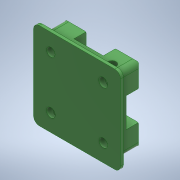
# Autodesk Inventor part: 071_0100_Base
Saved by Autodesk Inventor 2020 (Build 240168000, 168)
## iProperties
Created: 2018-07-06
Part Number: 071_0100_Base
Material: Generic
Document SubType Name: Modeling
Designer: deniz
Density: 1 g/cm^3
Appearance: Default
d_clamp_total: 51.477 mm
d_clamp_center: 25.739 mm
d_bottom_length: 52.400 mm
Author: deniz
Autodesk Inventor part; units mm, degrees
ref_plane "YZ Plane" through (0, 0, 0) normal (1, 0, 0) x (0, 1, 0)
ref_plane "XZ Plane" through (0, 0, 0) normal (0, 1, 0) x (-1, 0, 0)
ref_plane "XY Plane" through (0, 0, 0) normal (0, 0, 1) x (1, 0, 0)
sketch "Sketch1" plane through (0, 0, 0) normal (0, 1, 0) x (-1, 0, 0)
  line L0 (0, 0) -> (30, 0)
  line L1 (30, 0) -> (30, -30)
  line L2 (30, -30) -> (0, -30)
  line L3 (0, -30) -> (0, 0)
  line L4 (30, 0) -> (0, -30) construction
  line L5 (0, 0) -> (30, -30) construction
  line L6 (25.2, 0) -> (25.2, -4.8)
  line L7 (25.2, -4.8) -> (30, -4.8)
  line L8 (25.2, -25.2) -> (25.2, -30)
  line L9 (25.2, -25.2) -> (30, -25.2)
  line L10 (4.8, -25.2) -> (0, -25.2)
  line L11 (4.8, -25.2) -> (4.8, -30)
  line L12 (4.8, -4.8) -> (4.8, 0)
  line L13 (4.8, -4.8) -> (0, -4.8)
  line L14 (41.2, 11.2) -> (-11.2, 11.2)
  line L15 (-11.2, 11.2) -> (-11.2, -41.2)
  line L16 (-11.2, -41.2) -> (41.2, -41.2)
  line L17 (41.2, -41.2) -> (41.2, 11.2)
  circle A0 centre (33.2, 3.2) radius 5 construction
  line L18 (25.2, 0) -> (25.2, 11.2)
  line L19 (30, -4.8) -> (41.2, -4.8)
  line L20 (4.8, 0) -> (4.8, 11.2)
  line L21 (0, -4.8) -> (-11.2, -4.8)
  line L22 (0, -25.2) -> (-11.2, -25.2)
  line L23 (4.8, -30) -> (4.8, -41.2)
  line L24 (25.2, -30) -> (25.2, -41.2)
  line L25 (30, -25.2) -> (41.2, -25.2)
  line L26 (33.2, 3.2) -> (-3.2, -33.2) construction
  line L27 (33.2, 3.2) -> (-3.2, 3.2) construction
  line L28 (-3.2, 3.2) -> (-3.2, -33.2) construction
  line L29 (-3.2, -33.2) -> (33.2, -33.2) construction
  line L30 (33.2, -33.2) -> (33.2, 3.2) construction
  circle A1 centre (56.9794, 13.0498) radius 7.5
  arc A2 (58.5888, -1.0296) -> (56.9794, 13.0498) centre (33.2, 3.2) ccw construction
  arc A3 (62.0412, -1.6047) -> (60.213, 14.3892) centre (33.2, 3.2) ccw
  arc A4 (55.1364, -0.4544) -> (53.7459, 11.7104) centre (33.2, 3.2) ccw
  arc A5 (55.1364, -0.4544) -> (62.0412, -1.6047) centre (58.5888, -1.0296) ccw
  arc A6 (60.213, 14.3892) -> (53.7459, 11.7104) centre (56.9794, 13.0498) ccw
  line L31 (56.9794, 13.0498) -> (33.2, 3.2) construction
  point P0 (15, -15)
  dimension "d0" = 30
  dimension "d1" = 30
  dimension "d2" = 20.4
  dimension "d13" = 10
  dimension "d_clamp_total" = 51.4774
  dimension "d_clamp_center" = 25.7387
  dimension "d_bottom_length" = 52.4
  dimension "d52" = 8
  dimension "d53" = 8
  dimension "d54" = 8
  dimension "d55" = 8
  dimension "d56" = 8
  dimension "d58" = 15
  dimension "d59" = 7
  dimension "d61" = 22.5
  dimension "d62" = 25.7387
  dimension "d73" = 8
  dimension "d74" = 8
  constraints: 64 end point, 31 point on line, 10 perpendicular, 10 point on circle, 7 centre point, 6 coincident, 6 parallel, 4 tangent, 3 horizontal, 2 midpoint, 1 vertical
  measures "d0" distance of L1.end L2.end
  measures "d1" distance of L0.end L1.end
  measures "d2" distance between parallel lines of L9 L7
  measures "d13" diameter of A0
  measures "d_clamp_total" distance of L26.start L26.end
  measures "d_clamp_center" distance of point (15, -15) A0.centre
  measures "d_bottom_length" distance between parallel lines of L15 L17
  measures "d52" distance between parallel lines of L15 L28
  measures "d53" distance between parallel lines of L16 L29
  measures "d54" distance between parallel lines of L14 L27
  measures "d55" distance between parallel lines of L17 L30
  measures "d56" distance between parallel lines of L24 L30
  measures "d58" diameter of A1
  measures "d59" diameter of A5
  measures "d61" angle of L27 L31
  measures "d62" distance of L31.start L26.start
  measures "d73" distance from line of L26.end L23
  measures "d74" distance from line of L22 L26.end
extrude "Extrusion1" add sketch "Sketch1" along normal blind 2 contours L20 L14 L18 L0 | L0 L6 L7 L1 L9 L8 L2 L11 L10 L3 L13 L12 | L3 L22 L15 L21 | L19 L17 L25 L1 | L2 L24 L16 L23
extrude "Extrusion2" add sketch "Sketch1" along normal blind 12 contours L3 L21 L15 L14 L20 L0 | L0 L12 L13 L3 | L18 L14 L17 L19 L1 L0 | L0 L1 L7 L6 | L10 L11 L2 L3 | L3 L2 L23 L16 L15 L22 | L25 L17 L16 L24 L2 L1 | L1 L2 L8 L9
hole "Hole1" at (-33.2, 0, -33.2) at (3.2, 0, 3.2) direction (0, 1, 0) diameter 6.2 depth 20 tip angle 118 start extended yes
hole "Hole2" at (3.2, 0, -33.2) at (-33.2, 0, 3.2) direction (0, 1, 0) diameter 5.9 depth 20 tip angle 118 start extended yes
sketch "Sketch2" plane through (0, 12, 0) normal (0, 1, 0) x (1, 0, 0)
  circle A0 centre (-56.9794, -13.0498) radius 7.5 projected
  point P0 (0, 0)
extrude "Extrusion4" [suppressed]
sketch "Sketch3" plane through (-56.9794, 18, 13.0498) normal (0, 1, 0) x (1, 0, 0)
  circle A0 centre (60.1794, 46.2498) radius 2.95 projected
  circle A1 centre (23.7794, 9.8498) radius 2.95 projected
  circle A2 centre (23.7794, 46.2498) radius 3.1 projected
  circle A3 centre (60.1794, 9.8498) radius 3.1 projected
  line L0 (15.7794, 54.2498) -> (15.7794, 1.8498) projected
  line L1 (68.1794, 54.2498) -> (15.7794, 54.2498) projected
  line L2 (68.1794, 1.8498) -> (68.1794, 54.2498) projected
  line L3 (15.7794, 1.8498) -> (68.1794, 1.8498) projected
  arc A4 (1.8431, 13.5042) -> (-5.0618, 14.6545) centre (-1.6093, 14.0793) ccw projected
  arc A5 (-5.0618, 14.6545) -> (-3.2336, -1.3394) centre (23.7794, 9.8498) ccw projected
  arc A6 (1.8431, 13.5042) -> (3.2336, 1.3394) centre (23.7794, 9.8498) ccw projected
  arc A7 (-3.2336, -1.3394) -> (3.2336, 1.3394) centre (0, 0) ccw projected
  point P0 (56.9794, 13.0498)
extrude "Extrusion5" [suppressed]
fillet "Fillet5" [suppressed]
chamfer "TopChamfer1" distance 1.5 angle 45 16 edges at (-25.2, 12, 3.2) (-33.2, 12, -4.8) (-33.2, 12, -25.2) (-25.2, 12, -33.2) (-4.8, 12, -33.2) (3.2, 12, -25.2) (3.2, 12, -4.8) (-4.8, 12, 3.2) (-33.2, 12, 11.2) (-41.2, 12, 3.2) (-41.2, 12, -33.2) (-33.2, 12, -41.2) (3.2, 12, 11.2) (11.2, 12, 3.2) (11.2, 12, -33.2) (3.2, 12, -41.2)
fillet "Fillet1" radius 4 4 edges at (-41.2, 5.25, 11.2) (11.2, 5.25, 11.2) (11.2, 5.25, -41.2) (-41.2, 5.25, -41.2)
sketch "Sketch5" plane through (0, 0, 0) normal (0, -1, 0) x (1, 0, 0)
  circle A0 centre (3.2, -33.2) radius 2.95 projected
  circle A1 centre (-33.2, 3.2) radius 2.95 projected
  circle A2 centre (-33.2, -33.2) radius 3.1 projected
  circle A3 centre (3.2, 3.2) radius 3.1 projected
  arc A4 (-41.2, -37.2) -> (-37.2, -41.2) centre (-37.2, -37.2) ccw projected
  line L0 (7.2, -41.2) -> (-37.2, -41.2) projected
  arc A5 (7.2, -41.2) -> (11.2, -37.2) centre (7.2, -37.2) ccw projected
  line L1 (11.2, 7.2) -> (11.2, -37.2) projected
  arc A6 (11.2, 7.2) -> (7.2, 11.2) centre (7.2, 7.2) ccw projected
  line L2 (-37.2, 11.2) -> (7.2, 11.2) projected
  arc A7 (-37.2, 11.2) -> (-41.2, 7.2) centre (-37.2, 7.2) ccw projected
  line L3 (-41.2, -37.2) -> (-41.2, 7.2) projected
  line L4 (-3, 11.2) -> (-3, 31.2)
  line L5 (-3, 31.2) -> (7.2, 31.2)
  line L6 (7.2, 11.2) -> (7.2, 31.2) construction
  arc A8 (7.2, 31.2) -> (7.2, 11.2) centre (18.3803, 21.2) ccw
  line L7 (-15, 11.2) -> (-15, -41.2) construction
  point P0 (0, 0)
  dimension "d80" = 15
  dimension "d81" = 20
  dimension "d82" = 12
  constraints: 9 end point, 2 midpoint, 2 perpendicular, 2 point on circle, 1 centre point, 1 point on line, 1 vertical
  measures "d80" radius of A8
  measures "d81" distance of L4.start L4.end
  measures "d82" distance between parallel lines of L4 L7
ref_plane "Work Plane2" through (-15, 2, -4.8) normal (1, 0, 0) x (0, 0, -1)
ref_plane "Work Plane3" through (-4.8, 2, -15) normal (0, 0, -1) x (-1, 0, 0)
extrude "Holder" [suppressed]
fillet "Fillet6" [suppressed]
mirror "Mirror1" [suppressed]
mirror "Mirror2" [suppressed]
ref_plane "Work Plane1" through (-25.2, 0, -4.8) normal (0.7071068, 0, 0.7071068) x (0, 1, 0)
sketch "Sketch4" plane through (-25.2, 0, -4.8) normal (0.7071068, 0, 0.7071068) x (0, 1, 0)
  line L0 (12, 20.5061) -> (12, 11.3137) projected
  line L1 (12, 11.3137) -> (12, 20.5061) projected
  line L2 (12, 2.1213) -> (12, 11.3137) projected
  line L3 (12, 11.3137) -> (12, 2.1213) projected
  line L4 (12, 2.1213) -> (12, -1.8787)
  line L5 (12, -1.8787) -> (11, -1.8787)
  line L6 (11, -1.8787) -> (11, 24.5061)
  line L7 (11, 24.5061) -> (12, 24.5061)
  line L8 (12, 24.5061) -> (12, 20.5061)
  point P0 (0, -14.425)
  point P1 (8, 14.2637)
  point P2 (8, 8.3637)
  point P3 (12, 11.3137)
  dimension "d76" = 1
  dimension "d77" = 4
  dimension "d78" = 4
  constraints: 10 end point, 4 perpendicular, 1 point on line, 1 vertical
  measures "d76" distance between parallel lines of L0 L6
  measures "d77" distance from line of L0.start L7
  measures "d78" distance of L2.start L4.end
revolve "Revolution1Marker" cut sketch "Sketch4" angle 360 about axis through (-26.7, 12, -3.3) along (-0.7071068, 0, 0.7071068)
fillet "Orientation_Fillet2" radius 3 2 edges at (-25.2, 6.25, -4.8) (-25.45, 10.75, -4.55)
fillet "OverPrint_Fillet3" radius 1.5 17 edges at (-25.2, 6.25, -25.2) (-25.95, 11.25, -25.95) (-4.8, 6.25, -25.2) (-4.05, 11.25, -25.95) (-4.8, 6.25, -4.8) (-4.05, 11.25, -4.05) (9.8642, 11.8358, 9.8642) (9.8642, 11.8358, -39.8642) (10.45, 11.25, -25.95) (10.45, 11.25, -4.05) (-4.05, 11.25, 10.45) (-25.95, 11.25, 10.45) (-40.45, 11.25, -4.05) (-40.45, 11.25, -25.95) (-39.8642, 11.8358, -39.8642) (-25.95, 11.25, -40.45) (-4.05, 11.25, -40.45)
move faces "Move3" translate (0, -6, 0) faces at (-9.5854, 0, -20.3306)
sketch "Sketch7" plane through (-37.2, -6, -41.2) normal (0, -1, 0) x (1, 0, 0)
  circle A0 centre (40.4, 8) radius 2.95 projected
  circle A1 centre (4, 44.4) radius 2.95 projected
  circle A2 centre (4, 8) radius 3.1 projected
  circle A3 centre (40.4, 44.4) radius 3.1 projected
  arc A4 (-4, 4) -> (0, 0) centre (0, 4) ccw projected
  line L0 (44.4, 0) -> (0, 0) projected
  arc A5 (44.4, 0) -> (48.4, 4) centre (44.4, 4) ccw projected
  line L1 (48.4, 48.4) -> (48.4, 4) projected
  arc A6 (48.4, 48.4) -> (44.4, 52.4) centre (44.4, 48.4) ccw projected
  line L2 (0, 52.4) -> (44.4, 52.4) projected
  arc A7 (0, 52.4) -> (-4, 48.4) centre (0, 48.4) ccw projected
  line L3 (-4, 4) -> (-4, 48.4) projected
  line L4 (52.4, 56.4) -> (-8, 56.4)
  line L5 (-8, 56.4) -> (-8, -4)
  line L6 (-8, -4) -> (52.4, -4)
  line L7 (52.4, -4) -> (52.4, 56.4)
  point P0 (37.2, 41.2)
  dimension "d98" = 4
  dimension "d99" = 4
  dimension "d100" = 4
  dimension "d101" = 4
  constraints: 8 end point, 2 parallel, 1 horizontal, 1 perpendicular
  measures "d98" distance between parallel lines of L6 L0
  measures "d99" distance between parallel lines of L5 L3
  measures "d100" distance between parallel lines of L2 L4
  measures "d101" distance between parallel lines of L7 L1
extrude "Extrusion7" add sketch "Sketch7" against normal blind 2 contours L7 L6 L5 L4
fillet "Fillet8" radius 4 4 edges at (15.2, -5, 15.2) (-45.2, -5, 15.2) (15.2, -5, -45.2) (-45.2, -5, -45.2)
fillet "Fillet8" radius 2 8 edges at (10.0284, -4, 10.0284) (11.2, -4, -15) (10.0284, -4, -40.0284) (-15, -4, -41.2) (-40.0284, -4, -40.0284) (-41.2, -4, -15) (-40.0284, -4, 10.0284) (-15, -4, 11.2)
sketch "Sketch6" plane through (-25.2, 2, 11.2) normal (0, 0, 1) x (1, 0, 0)
  line L0 (36.4, 8.5) -> (36.4, 8.2158) projected
  line L1 (36.4, -4) -> (36.4, 8.5) projected
  line L2 (36.4, 8.5) -> (36.4, -4) projected
  line L3 (36.4, 8.2158) -> (36.4, 8.5) projected
  line L4 (36.4, 0) -> (36.4, 8.2158) projected
  line L5 (36.4, 0) -> (36.4, 8.2158) projected
  line L6 (20.4, 8.5) -> (20.4, 8.2158) projected
  line L7 (20.4, 0) -> (20.4, 8.5) projected
  line L8 (20.4, 0) -> (20.4, 8.2158) projected
  line L9 (32.4, 8.5) -> (21.4607, 8.5) projected
  line L10 (31.35, -8) -> (25.45, -8) projected
  line L11 (-5.05, -8) -> (-10.95, -8) projected
  line L12 (-4.9, -8) -> (-11.1, -8) projected
  line L13 (31.5, -8) -> (25.3, -8) projected
  line L14 (20.4, -2) -> (36.4, -2) construction
  point P0 (25.2, -2)
  point P1 (28.4, -2)
  constraints: 2 end point, 2 point on line, 1 midpoint, 1 perpendicular
hole "Hole3" at (3.2, 0, 11.2) direction (0, 0, -1) diameter 5.9 depth 14 start extended yes
pattern_circular "Circular Pattern1" count 2 over 360 about axis through (-15, 2, -15) along (0, 1, 0) of "Hole3"
equation "\"d53\" = d52"
equation "\"d62\" = d_clamp_center"
equation "\"d_bottom_frame\" = 4"
body "Solid1"
